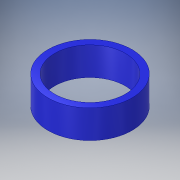
# Autodesk Inventor part: NoseCone_S3
Saved by Autodesk Inventor 2018 (Build 220112000, 112)
## iProperties
Created: 2017-10-02
Part Number: NoseCone_S3
Material: Generic
Document SubType Name: Modeling
Designer: Intel
Density: 1 g/cm^3
Appearance: Blue - Wall Paint - Glossy
Author: Intel
Autodesk Inventor part; units mm, degrees
ref_plane "YZ Plane" through (0, 0, 0) normal (1, 0, 0) x (0, 1, 0)
ref_plane "XZ Plane" through (0, 0, 0) normal (0, 1, 0) x (-1, 0, 0)
ref_plane "XY Plane" through (0, 0, 0) normal (0, 0, 1) x (1, 0, 0)
sketch "Sketch1" plane through (0, 0, 0) normal (0, 0, 1) x (1, 0, 0)
  line L0 (0, 0) -> (-39.6875, 0)
  line L1 (0, 0) -> (0, 127)
  arc A0 (0, 127) -> (-39.6875, 0) centre (313.5764, -40.6938) ccw
  line L2 (0, 0) -> (-37.7031, 0)
  line L3 (-37.7031, 0) -> (-37.7031, -25.4)
  line L4 (-37.7031, -25.4) -> (0, -25.4)
  line L5 (0, -25.4) -> (0, 0)
  line L6 (0, 63.5) -> (-26.4163, 63.5)
  line L7 (-20.0663, 63.5) -> (0, 63.5)
  line L8 (0, 63.5) -> (0, 44.45)
  line L9 (0, 44.45) -> (-20.0663, 44.45)
  line L10 (-20.0663, 44.45) -> (-20.0663, 63.5)
  line L11 (-20.0663, 44.45) -> (-20.0663, 0)
  line L12 (-20.0663, 0) -> (-31.75, 0)
  line L13 (-31.75, 0) -> (-31.75, -19.05)
  line L14 (-31.75, -19.05) -> (-20.0663, -19.05)
  line L15 (-20.0663, -19.05) -> (-20.0663, 0)
  line L16 (-31.75, -19.05) -> (-31.75, -25.4)
  dimension "d0" = 39.6875
  dimension "d1" = 127
  dimension "d3" = 355.6
  dimension "d5" = 37.7031
  dimension "d6" = 25.4
  dimension "d7" = 63.5
  dimension "d9" = 19.05
  dimension "d10" = 6.35
  dimension "d11" = 19.05
  dimension "d12" = 5.9531
  constraints: 34 end point, 6 parallel, 5 horizontal, 5 perpendicular, 4 point on line, 3 point on circle, 1 centre point, 1 midpoint, 1 vertical
  measures "d0" distance of L0.start L0.end
  measures "d1" distance of L0.start L1.end
  measures "d3" radius of A0
  measures "d5" distance of L4.end L3.end
  measures "d6" distance between parallel lines of L0 L4
  measures "d7" distance of L6.start L1.end
  measures "d9" distance of L7.end L8.end
  measures "d10" distance from line of L6.end L10
  measures "d11" distance of L13.end L12.end
  measures "d12" distance between parallel lines of L3 L13
revolve "Revolution1" add sketch "Sketch1" angle 360 about axis through (0, 0, 0) along (0, 1, 0) contours L13 L16 L4 L3 L0
body "Solid1"
